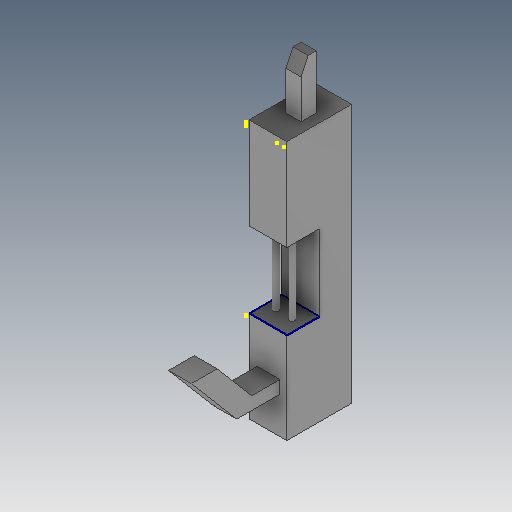
# Autodesk Inventor part: exploration cuboid
Saved by Autodesk Inventor 2021 (Build 250183000, 183)
## iProperties
Created: 2021-06-21
Part Number: exploration cuboid
Material: Silicon Nitride
Document SubType Name: Modeling
Designer: Lenovo
Density: 3.18 g/cm^3
Appearance: Chrome - Polished Black
Author: Lenovo
Autodesk Inventor part; units mm, degrees
ref_plane "YZ Plane" through (0, 0, 0) normal (1, 0, 0) x (0, 1, 0)
ref_plane "XZ Plane" through (0, 0, 0) normal (0, 1, 0) x (-1, 0, 0)
ref_plane "XY Plane" through (0, 0, 0) normal (0, 0, 1) x (1, 0, 0)
sketch "Sketch1" plane through (0, 0, 0) normal (1, 0, 0) x (0, 1, 0)
  line L0 (7.9725, -6.9898) -> (-601.6275, -6.9898)
  line L1 (-601.6275, -6.9898) -> (-601.6275, -159.3898)
  line L2 (-601.6275, -159.3898) -> (7.9725, -159.3898)
  line L3 (7.9725, -159.3898) -> (7.9725, -6.9898)
  point P0 (0, 0)
  dimension "d0" = 609.6
  dimension "d1" = 152.4
  constraints: 8 end point, 2 parallel, 1 horizontal, 1 perpendicular
  measures "d0" distance of L2.end L1.end
  measures "d1" distance of L1.end L0.end
extrude "Extrusion1" add sketch "Sketch1" along normal blind 88.9
sketch "Sketch2" plane through (0, -601.6275, -6.9898) normal (0, 0, 1) x (1, 0, 0)
  line L0 (0, 0) -> (0, 609.6) projected
  line L1 (0, 609.6) -> (0, 393.7)
  line L2 (0, 0) -> (88.9, 0) projected
  line L3 (0, 0) -> (0, 215.9)
  line L4 (88.9, 0) -> (88.9, 609.6) projected
  line L5 (0, 393.7) -> (88.9, 393.7)
  line L6 (88.9, 393.7) -> (88.9, 215.9)
  line L7 (88.9, 215.9) -> (0, 215.9)
  line L8 (0, 215.9) -> (0, 393.7)
  line L9 (0, 393.7) -> (0, 215.9)
  point P0 (0, 601.6275)
  point P1 (0, 215.9)
  dimension "d4" = 215.9
  dimension "d5" = 215.9
  constraints: 14 end point, 3 point on line, 2 parallel, 1 collinear, 1 horizontal, 1 perpendicular
  measures "d4" distance of L0.end L1.end
  measures "d5" distance of L0.start L3.end
extrude "Extrusion2" cut sketch "Sketch2" against normal blind 76.2 contours L0 L5 L4 L7
sketch "Sketch3" plane through (88.9, 0, 0) normal (1, 0, 0) x (0, 0, -1)
  point P0 (0, 0)
sketch "Sketch4" plane through (0, -601.6275, -6.9898) normal (0, 0, 1) x (1, 0, 0)
  line L0 (18.9312, 116.4608) -> (72.6429, 116.4608)
  line L1 (72.6429, 116.4608) -> (72.6429, 86.5231)
  line L2 (72.6429, 86.5231) -> (18.9312, 86.5231)
  line L3 (18.9312, 86.5231) -> (18.9312, 116.4608)
  point P0 (0, 601.6275)
  constraints: 8 end point, 2 parallel, 1 horizontal, 1 perpendicular
extrude "Extrusion3" add sketch "Sketch4" along normal blind 101.6
sketch "Sketch5" plane through (72.6429, -515.1044, -6.9898) normal (1, 0, 0) x (0, 0, -1)
  line L0 (-101.6, 0) -> (-66.3848, 29.9377)
  line L1 (0, 29.9377) -> (-101.6, 29.9377) projected
  line L2 (-101.6, 0) -> (-101.6, 29.9377) projected
  line L3 (-101.6, 0) -> (-101.6, 29.9377)
  point P0 (-6.9898, 515.1044)
  constraints: 4 end point, 1 collinear, 1 point on line
extrude "Extrusion4" cut sketch "Sketch5" against normal through all
sketch "Sketch6" plane through (18.9312, -515.1044, 94.6102) normal (0, 0.7618887, 0.647708) x (1, 0, 0)
  line L0 (0, 46.221) -> (53.7117, 46.221) projected
  line L1 (53.7117, 77.4079) -> (53.7117, 0) projected
  line L2 (0, 46.221) -> (53.7117, 46.221)
  line L3 (53.7117, 46.221) -> (53.7117, 0)
  line L4 (53.7117, 0) -> (0, 0)
  line L5 (0, 0) -> (0, 46.221)
  point P0 (-18.9312, 405.7197)
  constraints: 8 end point, 2 parallel, 1 horizontal, 1 perpendicular
extrude "Extrusion5" add sketch "Sketch6" along normal blind 165.1
sketch "Sketch7" plane through (72.6429, -515.1044, -6.9898) normal (1, 0, 0) x (0, 0, -1)
  point P0 (-6.9898, 515.1044)
sketch "Sketch8" plane through (72.6429, -515.1044, -6.9898) normal (1, 0, 0) x (0, 0, -1)
  line L0 (-173.3214, 155.7255) -> (-208.5366, 125.7878) projected
  line L1 (-208.5366, 125.7878) -> (-147.8703, 125.7878)
  line L2 (-66.3848, 29.9377) -> (-173.3214, 155.7255) projected
  line L3 (-173.3214, 155.7255) -> (-208.5366, 125.7878)
  line L4 (-147.8703, 125.7878) -> (-173.3214, 155.7255)
  point P0 (-6.9898, 515.1044)
  constraints: 6 end point, 1 horizontal, 1 perpendicular, 1 point on line
extrude "Extrusion6" cut sketch "Sketch8" against normal through all
sketch "Sketch9" plane through (72.6429, -389.3166, 201.5467) normal (0, 1, 0) x (1, 0, 0)
  point P0 (-72.6429, 201.5467)
sketch "Sketch10" plane through (0, -385.7275, -6.9898) normal (0, 1, 0) x (1, 0, 0)
  point P0 (0, -6.9898)
sketch "Sketch11" plane through (0, -385.7275, -6.9898) normal (0, 1, 0) x (1, 0, 0)
  point P0 (0, -6.9898)
sketch "Sketch12" plane through (0, -385.7275, -6.9898) normal (0, 1, 0) x (1, 0, 0)
  point P0 (0, -6.9898)
sketch "Sketch13" plane through (0, 0, 0) normal (-1, 0, 0) x (0, 0, 1)
  point P0 (0, 0)
sketch "Sketch14" plane through (0, -385.7275, -6.9898) normal (0, 1, 0) x (1, 0, 0)
  line L0 (88.9, 76.2) -> (0, 76.2) projected
  line L1 (0, 0) -> (0, 76.2) projected
  line L2 (88.9, 76.2) -> (0, 76.2)
  line L3 (88.9, 76.2) -> (88.9, 0) projected
  line L4 (0, 76.2) -> (88.9, 76.2)
  line L5 (88.9, 76.2) -> (0, 76.2)
  line L6 (0, 76.2) -> (0, 0)
  line L7 (0, 0) -> (88.9, 0)
  line L8 (88.9, 0) -> (88.9, 76.2)
  point P0 (0, -6.9898)
  constraints: 12 end point, 2 horizontal, 2 parallel, 2 perpendicular
sketch "Sketch15" plane through (0, -385.7275, -6.9898) normal (0, 1, 0) x (1, 0, 0)
  line L0 (88.9, 76.2) -> (88.9, 0) projected
  line L1 (88.9, 38.1) -> (0, 38.1)
  line L2 (0, 0) -> (0, 76.2) projected
  line L3 (88.9, 76.2) -> (0, 76.2)
  circle A0 centre (63.5, 38.1) radius 6.35
  circle A1 centre (25.4, 38.1) radius 6.35
  point P0 (0, -6.9898)
  dimension "d20" = 12.7
  dimension "d21" = 12.7
  constraints: 4 coincident, 4 end point, 2 centre point, 2 midpoint, 2 point on line, 1 perpendicular
  measures "d20" diameter of A0
  measures "d21" diameter of A1
extrude "Extrusion7" add sketch "Sketch15" along normal blind 177.8 contours A0 L1 | L1 A0 | A1 L1 | L1 A1
sketch "Sketch16" plane through (0, 7.9725, -6.9898) normal (0, 1, 0) x (1, 0, 0)
  line L0 (29.6959, 92.8158) -> (65.2559, 92.8158)
  line L1 (65.2559, 92.8158) -> (65.2559, 57.2558)
  line L2 (65.2559, 57.2558) -> (29.6959, 57.2558)
  line L3 (29.6959, 57.2558) -> (29.6959, 92.8158)
  point P0 (0, -6.9898)
  dimension "d24" = 35.56
  dimension "d25" = 35.56
  constraints: 8 end point, 2 parallel, 1 horizontal, 1 perpendicular
  measures "d24" distance of L1.end L2.end
  measures "d25" distance of L0.end L1.end
extrude "Extrusion8" add sketch "Sketch16" along normal blind 127
sketch "Sketch17" plane through (29.6959, 7.9725, -64.2457) normal (0, 0, 1) x (1, 0, 0)
  line L0 (0, 127) -> (35.56, 127) projected
  line L1 (35.56, 0) -> (35.56, 127) projected
  line L2 (0, 127) -> (35.56, 127)
  line L3 (35.56, 127) -> (35.56, 91.44)
  line L4 (35.56, 91.44) -> (0, 91.44)
  line L5 (0, 91.44) -> (0, 127)
  point P0 (-29.6959, -7.9725)
  dimension "d28" = 35.56
  constraints: 8 end point, 2 parallel, 1 horizontal, 1 perpendicular, 1 point on line
  measures "d28" distance of L2.end L3.end
extrude "Extrusion9" add sketch "Sketch17" along normal blind 127
sketch "Sketch18" plane through (65.2559, 7.9725, -64.2457) normal (1, 0, 0) x (0, 0, -1)
  line L0 (0, 91.44) -> (-127, 91.44) projected
  line L1 (-64.2457, 91.44) -> (-45.72, 127)
  line L2 (35.56, 127) -> (-127, 127) projected
  line L3 (-45.72, 127) -> (-127, 127)
  line L4 (-127, 127) -> (-127, 91.44) projected
  line L5 (-127, 91.44) -> (-64.2457, 91.44)
  line L6 (-127, 127) -> (-127, 91.44)
  line L7 (35.56, 127) -> (-127, 127) projected
  line L8 (0, 127) -> (-14.8626, 91.44)
  line L9 (-64.2457, 91.44) -> (-14.8626, 91.44)
  line L10 (-14.8626, 91.44) -> (0, 127)
  line L11 (-45.72, 127) -> (-127, 127)
  line L12 (0, 127) -> (-49.9714, 127)
  point P0 (-64.2457, -7.9725)
  constraints: 18 end point, 4 point on line, 3 collinear, 1 midpoint, 1 parallel, 1 perpendicular
extrude "Extrusion10" cut sketch "Sketch18" against normal through all contours L0 L4 L2 L1
sketch "Sketch19" plane through (65.2559, 7.9725, -64.2457) normal (1, 0, 0) x (0, 0, -1)
  line L0 (0, 91.44) -> (-64.2457, 91.44) projected
  line L1 (-32.1228, 91.44) -> (-14.9944, 127)
  line L2 (35.56, 127) -> (-45.72, 127) projected
  line L3 (-32.1228, 91.44) -> (-64.2457, 91.44)
  line L4 (-64.2457, 91.44) -> (-45.72, 127) projected
  line L5 (-64.2457, 91.44) -> (-45.72, 127)
  line L6 (-45.72, 127) -> (-14.9944, 127)
  point P0 (-64.2457, -7.9725)
  constraints: 8 end point, 1 collinear, 1 horizontal, 1 midpoint, 1 parallel, 1 point on line
extrude "Extrusion11" cut sketch "Sketch19" against normal through all
sketch "Sketch20" plane through (65.2559, 7.9725, -64.2457) normal (1, 0, 0) x (0, 0, -1)
  line L0 (35.56, 127) -> (-14.9944, 127) projected
  line L1 (-0.2658, 127) -> (-21.0098, 91.44)
  line L2 (0, 91.44) -> (-32.1228, 91.44) projected
  line L3 (-21.0098, 91.44) -> (-32.1228, 91.44)
  line L4 (-32.1228, 91.44) -> (-14.9944, 127) projected
  line L5 (-32.1228, 91.44) -> (-14.9944, 127)
  line L6 (-14.9944, 127) -> (-0.2658, 127)
  point P0 (-64.2457, -7.9725)
  constraints: 8 end point, 2 point on line, 1 collinear, 1 horizontal, 1 parallel
extrude "Extrusion12" cut sketch "Sketch20" against normal through all
sketch "Sketch21" plane through (0, 7.9725, -6.9898) normal (0, 1, 0) x (1, 0, 0)
  point P0 (0, -6.9898)
sketch "Sketch22" plane through (65.2559, 7.9725, -64.2457) normal (1, 0, 0) x (0, 0, -1)
  line L0 (-0.2658, 127) -> (-21.0098, 91.44) projected
  line L1 (-21.0098, 91.44) -> (-0.2658, 127)
  line L2 (-0.2658, 127) -> (16.5705, 127)
  line L3 (35.56, 127) -> (-0.2658, 127) projected
  line L4 (0, 0) -> (0, 91.44) projected
  line L5 (0, 91.44) -> (16.5705, 127)
  line L6 (0, 91.44) -> (-21.0098, 91.44) projected
  line L7 (0, 91.44) -> (-21.0098, 91.44)
  point P0 (-64.2457, -7.9725)
  constraints: 8 end point, 2 collinear, 1 point on line
extrude "Extrusion13" cut sketch "Sketch22" against normal through all
body "Solid1"
